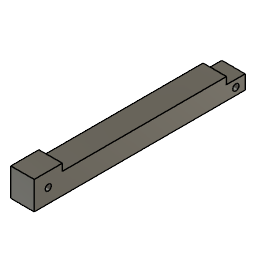
Arm v1 (Autodesk Fusion 360 design; units mm, degrees)
Autodesk Fusion 360 part; units mm, degrees
sketch "Sketch1" plane through (0, 0, 0) normal (1, 0, 0) x (0, 1, 0)
  line L0 (0, 0) -> (0, 24)
  line L1 (0, 24) -> (24, 24)
  line L2 (24, 24) -> (24, 18)
  line L3 (24, 18) -> (164, 18)
  line L4 (164, 18) -> (164, 12)
  line L5 (164, 12) -> (180, 12)
  line L6 (180, 12) -> (180, 0)
  line L7 (0, 0) -> (180, 0)
  circle A0 centre (12, 12) radius 2.6
  circle A1 centre (172, 6) radius 2.65
  dimension "d6" = 24
  dimension "d7" = 24
  dimension "d8" = 6
  dimension "d9" = 140
  dimension "d10" = 6
  dimension "d11" = 16
  dimension "d12" = 12
  dimension "d15" = 5.2
  dimension "d18" = 5.3
  constraint coincident L0.start L7.start
  constraint vertical L0
  constraint perpendicular L0 L1
  constraint perpendicular L1 L2
  constraint perpendicular L2 L3
  constraint perpendicular L3 L4
  constraint perpendicular L4 L5
  constraint perpendicular L5 L6
  measures "d6" distance of L0.start L0.end
  measures "d7" distance of L0.end L1.end
  measures "d8" distance of L1.end L2.end
  measures "d9" distance of L2.end L3.end
  measures "d10" distance of L3.end L4.end
  measures "d11" distance of L4.end L5.end
  measures "d12" distance of L5.end L6.end
  measures "d15" diameter of A0
  measures "d18" diameter of A1
extrude "Extrude1" add sketch "Sketch1" along normal mid plane 20
